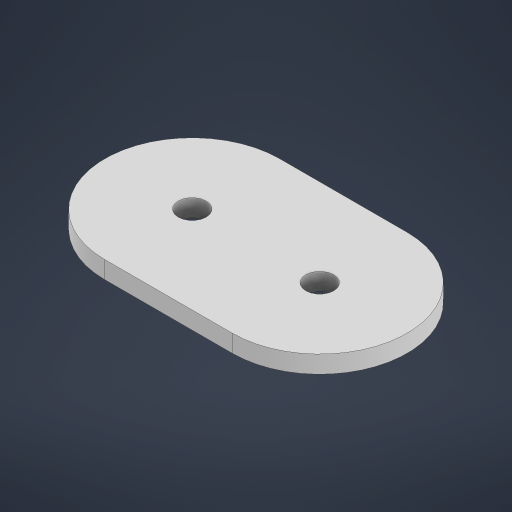
# Autodesk Inventor part: hinge
Saved by Autodesk Inventor 2024 (Build 280153000, 153)
## iProperties
Created: 2025-01-02
Part Number: hinge
Material: Generic
Document SubType Name: Modeling
Designer: turbo
Density: 1 g/cm^3
Appearance: Default
Author: turbo
Autodesk Inventor part; units mm, degrees
ref_plane "YZ Plane" through (0, 0, 0) normal (1, 0, 0) x (0, 1, 0)
ref_plane "XZ Plane" through (0, 0, 0) normal (0, 1, 0) x (-1, 0, 0)
ref_plane "XY Plane" through (0, 0, 0) normal (0, 0, 1) x (1, 0, 0)
sketch "Sketch1" plane through (0, 0, 0) normal (0, 1, 0) x (-1, 0, 0)
  arc A0 (13.9253, -19.1836) -> (13.9253, 18.9664) centre (13.9253, -0.1086) ccw
  arc A1 (-13.9253, 18.9664) -> (-13.9253, -19.1836) centre (-13.9253, -0.1086) ccw
  line L0 (33, 0) -> (-33, 0) construction
  line L1 (13.9253, 18.9664) -> (-13.9253, 18.9664)
  line L2 (14.2135, -19.1836) -> (-13.9253, -19.1836)
  line L3 (-13.9253, -0.1086) -> (-13.9253, 18.9664) construction
  line L4 (-13.9253, -0.1086) -> (-13.9253, -19.1836) construction
  line L5 (13.9253, 18.9664) -> (13.9253, -19.1836) construction
  circle A2 centre (13.9253, -0.1086) radius 3.05
  circle A3 centre (-13.9253, -0.1086) radius 3.05
  point P0 (0, 0)
  point P1 (0, 0)
  dimension "d0" = 38.15
  dimension "d1" = 66
  dimension "d4" = 27.8506
  dimension "d7" = 6.1
  constraints: 12 end point, 6 point on circle, 4 centre point, 4 tangent, 3 coincident, 2 equal radius, 2 vertical, 1 collinear, 1 horizontal, 1 horizontal alignment, 1 midpoint, 1 point on line
  measures "d0" diameter of A0
  measures "d1" distance of L0.start L0.end
  measures "d4" distance between parallel lines of L4 L5
  measures "d7" diameter of A3
extrude "Extrusion1" add sketch "Sketch1" along normal blind 3.8
body "Solid1"
